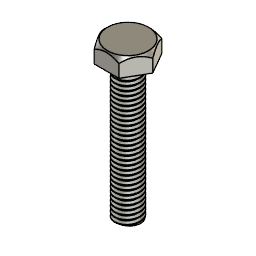
smartie_hopper_mechanism (Autodesk Fusion 360 archive; units mm, degrees)
design "M6 32 mm Hex Bolt"
part number: 2026-04-25-09-17-42-437
Autodesk Fusion 360 part; units mm, degrees
sketch "Thread" plane through (0, 0, 0) normal (0, 0, 1) x (1, 0, 0)
  circle A0 centre (0, 0) radius 3
  dimension "d2" = 6
  constraint coincident A0.centre origin
  measures "d2" diameter of A0
extrude "Extrude1" add sketch "Thread" along normal blind 32
sketch "Head" plane through (0, 0, 32) normal (0, 0, 1) x (-1, 0, 0)
  circle A0 centre (0, 0) radius 3
  line L0 (2.8868, -5) -> (5.7735, 0)
  line L1 (5.7735, 0) -> (2.8868, 5)
  line L2 (2.8868, 5) -> (-2.8868, 5)
  line L3 (-2.8868, 5) -> (-5.7735, 0)
  line L4 (-5.7735, 0) -> (-2.8868, -5)
  line L5 (-2.8868, -5) -> (2.8868, -5)
  dimension "d10" = 10
  constraint coincident A0.centre origin
  measures "d10" distance of L2 L5
extrude "Extrude2" add sketch "Head" along normal blind 4 contours A0 | L0 L1 L2 L3 L4 L5
thread "Thread1" "ISO Metric profile 6.0 M6x1 M6x1 6g" major diameter 5.884 minor diameter 4.7435 pitch 1 angle 60 modelled right hand crest width 0.1444 on face at (2.9963, -0.1495, 21.3333) crest through (2.942, 0, -0.25)
sketch "Head fillet" plane through (0, 0, 0) normal (0, 1, 0) x (1, 0, 0)
  line L0 (2.8868, -32) -> (5.7735, -32)
  line L1 (5.7735, -32) -> (5.7735, -36)
  line L2 (5.7735, -36) -> (2.8868, -36)
  line L3 (2.8868, -36) -> (2.8868, -32)
  line L4 (-5.7735, -32) -> (-2.8868, -32)
  line L5 (-2.8868, -32) -> (-2.8868, -36)
  line L6 (-2.8868, -36) -> (-5.7735, -36)
  line L7 (-5.7735, -36) -> (-5.7735, -32)
  line L8 (-2.8868, -32) -> (2.8868, -32)
  line L9 (2.8868, -32) -> (2.8868, -36)
  line L10 (2.8868, -36) -> (-2.8868, -36)
  line L11 (-2.8868, -36) -> (-2.8868, -32)
  line L12 (5.7735, -36) -> (4.7735, -36)
  line L13 (5.7735, -36) -> (5.7735, -35)
  line L14 (4.7735, -36) -> (5.7735, -35)
  dimension "d14" = 1
  dimension "d15" = 1
  constraint coincident L1.end L2.start
  constraint perpendicular L1 L12
  constraint perpendicular L2 L13
  measures "d14" distance of L1.end L12.end
  measures "d15" distance of L1.end L13.end
revolve "Revolve1" cut sketch "Head fillet" angle 360 about axis through (0, 0, 1.75) along (0, 0, 1) contours L1 L2 L12 L13 L14
equation "diameter = 6 mm" comment "An M6 hex bolt has a diameter of 6 mm."
equation "d2 = diameter"
equation "thread_height = 32 mm" comment "The length of the M6 hex bolt (excluding the head)."
equation "d4 = thread_height"
equation "head_height = 4 mm" comment "An M6 hex bolt has a head thickness of 4 mm."
equation "width_across_flats = 10 mm" comment "An M6 hex bolt has a width across the flats of 10 mm."
equation "d10 = width_across_flats"
equation "d11 = head_height"
equation "chamfer_side_length = 1 mm" comment "Chamfer on the top of the hex bolt head."
equation "d14 = chamfer_side_length"
equation "d15 = chamfer_side_length"
named bodies: "M6 32 mm Hex Bolt"

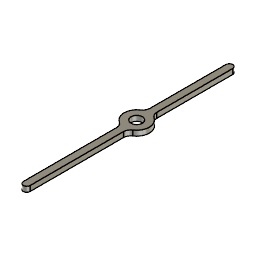
design "Mixer Arm"
part number: 2026-05-20-12-12-58-237
Autodesk Fusion 360 part; units mm, degrees
sketch "Mixer arm" plane through (0, 0, 0) normal (0, 0, 1) x (1, 0, 0)
  circle A0 centre (0, 0) radius 7.25
  circle A1 centre (0, 0) radius 3.25
  line L0 (-2, 55.25) -> (2, 55.25)
  line L1 (2, 55.25) -> (2, 3.25)
  line L2 (2, 3.25) -> (-2, 3.25)
  line L3 (-2, 3.25) -> (-2, 55.25)
  line L4 (-2, -3.25) -> (2, -3.25)
  line L5 (2, -3.25) -> (2, -65.25)
  line L6 (2, -65.25) -> (-2, -65.25)
  line L7 (-2, -65.25) -> (-2, -3.25)
  line L8 (-2, -7.25) -> (2, -7.25)
  line L9 (-2, 7.25) -> (2, 7.25)
  dimension "d3" = 6.5
  dimension "d5" = 14.5
  dimension "d6" = 2
  dimension "d7" = 2
  dimension "d8" = 2
  dimension "d9" = 2
  dimension "d14" = 58
  dimension "d15" = 48
  constraint coincident A0.centre A1.centre
  constraint concentric A0 A1
  constraint horizontal L0
  constraint vertical L1
  constraint horizontal L2
  constraint vertical L3
  constraint horizontal L4
  constraint vertical L5
  constraint horizontal L6
  constraint vertical L7
  constraint tangent A1 L2
  constraint tangent A1 L4
  constraint coincident L7 L8.start
  constraint coincident L5 L8.end
  constraint perpendicular L5 L8
  constraint tangent A0 L8
  constraint coincident L1 L9.end
  constraint perpendicular L1 L9
  constraint tangent A0 L9
  measures "d3" diameter of A1
  measures "d5" diameter of A0
  measures "d6" distance of A0.centre L1
  measures "d7" distance of A0.centre L3
  measures "d8" distance of A0.centre L7
  measures "d9" distance of A0.centre L5
  measures "d14" distance of L6 L8
  measures "d15" distance of L0 L9
extrude "Extrude1" add sketch "Mixer arm" along normal blind 3 contours A0 A1 L1 L2 L4 L5 | A0 L1 L2 L3 | A0 L1 L9 | A0 L5 L8 | A0 L4 L5 L7 | A0 L3 L9 | L0 L1 L3 L9 | A0 L7 L8 | L5 L6 L7 L8 | A0 A1 L2 L3 L4 L7
fillet "Fillet1" radius 4 4 edges at (2, -6.9687, 1.5) (2, 6.9687, 1.5) (-2, 6.9687, 1.5) (-2, -6.9687, 1.5)
fillet "Fillet2" radius 2 4 edges at (2, 55.25, 1.5) (-2, 55.25, 1.5) (-2, -65.25, 1.5) (2, -65.25, 1.5)
equation "stainless_steel_thickness = 3 mm" comment "The thickness of the 316 stainless steel sheets to laser cut."
equation "hole_diameter = 6.5 mm"
equation "d3 = hole_diameter"
equation "arm_thickness = 4 mm"
equation "d5 = hole_diameter + 2 * arm_thickness"
equation "d6 = arm_thickness / 2"
equation "d7 = arm_thickness / 2"
equation "d8 = arm_thickness / 2"
equation "d9 = arm_thickness / 2"
equation "d10 = stainless_steel_thickness"
equation "arm_length_front = 58 mm"
equation "arm_length_back = 48 mm"
equation "d14 = arm_length_front"
equation "d15 = arm_length_back"
equation "d17 = arm_thickness"
equation "d19 = arm_thickness / 2"
named bodies: "Mixer arm"

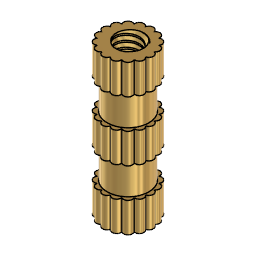
design "M2 10 mm Threaded Brass Insert"
part number: 2026-06-20-09-24-02-047
Autodesk Fusion 360 part; units mm, degrees
sketch "Brass thread outline" plane through (0, 0, 0) normal (0, 0, 1) x (1, 0, 0)
  circle A0 centre (0, 0) radius 1.4
  dimension "d4" = 2.8
  constraint coincident A0.centre origin
  measures "d4" diameter of A0
extrude "Extrude1" add sketch "Brass thread outline" along normal blind 10
sketch "Ridges" plane through (0, 0, 10) normal (0, 0, 1) x (-1, 0, 0)
  circle A0 centre (0, 0) radius 1.4
  circle A1 centre (0, 0) radius 1.7
  circle A2 centre (-0.0001, -1.4) radius 0.3
  circle A3 centre (0.5357, -1.2935) radius 0.3
  circle A4 centre (0.9899, -0.99) radius 0.3
  circle A5 centre (1.2934, -0.5358) radius 0.3
  circle A6 centre (1.4, -0.0001) radius 0.3
  circle A7 centre (1.2935, 0.5357) radius 0.3
  circle A8 centre (0.99, 0.9899) radius 0.3
  circle A9 centre (0.5358, 1.2934) radius 0.3
  circle A10 centre (0.0001, 1.4) radius 0.3
  circle A11 centre (-0.5357, 1.2935) radius 0.3
  circle A12 centre (-0.9899, 0.99) radius 0.3
  circle A13 centre (-1.2934, 0.5358) radius 0.3
  circle A14 centre (-1.4, 0.0001) radius 0.3
  circle A15 centre (-1.2935, -0.5357) radius 0.3
  circle A16 centre (-0.99, -0.9899) radius 0.3
  circle A17 centre (-0.5358, -1.2934) radius 0.3
  dimension "d8" = 3.4
  dimension "d29" = 0.0001
  dimension "d31" = 360
  constraint coincident A0.centre A1.centre
  constraint coincident A0 A2.centre
  constraint tangent A1 A2
  measures "d8" diameter of A1
  measures "d29" horizontal distance of A0.centre A2.centre
extrude "Extrude2" add sketch "Ridges" against normal blind 2 contours A0 A5 A6 A7 | A0 A5 A6 A7 | A0 A6 A7 | A0 A6 A7 | A0 A5 A6 | A0 A5 A6 | A0 A6 A7 A8 | A0 A6 A7 A8 | A2 A3 A4 A5 A6 A7 A8 A9 A10 A11 A12 A13 A14 A15 A16 A17 | A0 A4 A5 A6 | A0 A4 A5 A6 | A0 A7 A8 | A0 A7 A8 | A0 A7 A8 A9 | A0 A4 A5 | A0 A4 A5 | A0 A3 A4 A5 | A0 A7 A8 A9 | A0 A8 A9 A10 | A0 A8 A9 | A0 A3 A4 A5 | A0 A2 A3 A4 | A0 A3 A4 | A0 A8 A9 | A0 A8 A9 A10 | A0 A9 A10 A11 | A0 A9 A10 | A0 A3 A4 | A0 A2 A3 A17 | A0 A2 A3 | A0 A2 A3 A4 | A0 A9 A10 | A0 A9 A10 A11 | A0 A10 A11 A12 | A0 A10 A11 | A0 A2 A3 | A0 A2 A17 | A0 A2 A16 A17 | A0 A2 A3 A17 | A0 A10 A11 | A0 A10 A11 A12 | A0 A11 A12 A13 | A0 A11 A12 | A0 A2 A16 A17 | A0 A2 A17 | A0 A15 A16 A17 | A0 A16 A17 | A0 A11 A12 | A0 A11 A12 A13 | A0 A16 A17 | A0 A15 A16 A17 | A0 A12 A13 | A0 A12 A13 | A0 A12 A13 A14 | A0 A14 A15 A16 | A0 A15 A16 | A0 A15 A16 | A0 A12 A13 A14 | A0 A14 A15 A16 | A0 A13 A14 | A0 A13 A14 | A0 A13 A14 A15 | A0 A13 A14 A15 | A0 A14 A15 | A0 A14 A15
pattern_linear "R-Pattern1" count 3 spacing 4 along (0, 0, -1) of "Extrude2"
sketch "Thread hole" plane through (0, 0, 10) normal (0, 0, 1) x (-1, 0, 0)
  circle A0 centre (0, 0) radius 1
  arc A1 (0.292, -1.4685) -> (0.8317, -1.2449) centre (0.5357, -1.2935) ccw
  arc A2 (0.8317, -1.2449) -> (1.2448, -0.8319) centre (0.9899, -0.99) ccw
  arc A3 (1.2448, -0.8319) -> (1.4684, -0.2922) centre (1.2934, -0.5358) ccw
  arc A4 (1.4684, -0.2922) -> (1.4685, 0.292) centre (1.4, -0.0001) ccw
  arc A5 (1.4685, 0.292) -> (1.2449, 0.8317) centre (1.2935, 0.5357) ccw
  arc A6 (1.2449, 0.8317) -> (0.8319, 1.2448) centre (0.99, 0.9899) ccw
  arc A7 (0.8319, 1.2448) -> (0.2922, 1.4684) centre (0.5358, 1.2934) ccw
  arc A8 (0.2922, 1.4684) -> (-0.292, 1.4685) centre (0.0001, 1.4) ccw
  arc A9 (-0.292, 1.4685) -> (-0.8317, 1.2449) centre (-0.5357, 1.2935) ccw
  arc A10 (-0.8317, 1.2449) -> (-1.2448, 0.8319) centre (-0.9899, 0.99) ccw
  arc A11 (-1.2448, 0.8319) -> (-1.4684, 0.2922) centre (-1.2934, 0.5358) ccw
  arc A12 (-1.4684, 0.2922) -> (-1.4685, -0.292) centre (-1.4, 0.0001) ccw
  arc A13 (-1.4685, -0.292) -> (-1.2449, -0.8317) centre (-1.2935, -0.5357) ccw
  arc A14 (-1.2449, -0.8317) -> (-0.8319, -1.2448) centre (-0.99, -0.9899) ccw
  arc A15 (-0.8319, -1.2448) -> (-0.2922, -1.4684) centre (-0.5358, -1.2934) ccw
  arc A16 (-0.2922, -1.4684) -> (0.292, -1.4685) centre (-0.0001, -1.4) ccw
  dimension "d11" = 2
  constraint coincident A0.centre origin
  measures "d11" diameter of A0
extrude "Extrude3" cut sketch "Thread hole" against normal blind 10 contours A0
thread "Thread1" "ISO Metric profile 2.0 M2x0.4 M2x0.4 6H" major diameter 2.074 minor diameter 1.623 pitch 0.4 angle 60 modelled right hand crest width 0.1065 on face at (-0.9988, 0.0498, 3.3333) crest through (-0.8115, 0, 9.9)
equation "outer_diameter = 2.8 mm" comment "The outer diameter of the non-ridged parts."
equation "hole_diameter = 2 mm" comment "The thread diameter of the brass insert. 2 mm for this M2 insert."
equation "height = 10 mm" comment "The height of the brass thread insert. 10 mm for this model."
equation "d4 = outer_diameter"
equation "d5 = height"
equation "ridge_diameter = 3.4 mm" comment "The outer diameter of the ridged parts."
equation "d8 = ridge_diameter"
equation "d9 = -ridge_height"
equation "d11 = hole_diameter"
equation "d12 = -height"
equation "number_of_ridges = 3" comment "The number of ridges to have along the outside."
equation "d23 = number_of_ridges"
equation "d25 = -ridge_pattern_length"
equation "ridge_pattern_length = height - ridge_height" comment "The distance to use for the rectangular pattern that repeats the ridges."
equation "ridge_height = 2 mm" comment "The height of the individual ridges."
named bodies: "M2 10 mm Threaded Brass Insert"

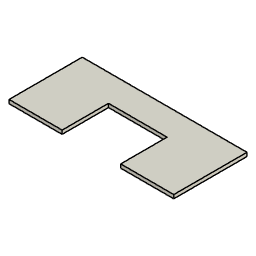
design "Colour Detection Mechanism Top Panel"
part number: 2025-05-13-09-48-31-121
Autodesk Fusion 360 part; units mm, degrees
sketch "Sorting Mechanism Top Panel" plane through (0, 0, 0) normal (0, 0, 1) x (1, 0, 0)
  line L0 (0, 0) -> (270, 0)
  line L1 (270, 0) -> (270, 120)
  line L2 (270, 120) -> (0, 120)
  line L3 (0, 120) -> (0, 0)
  dimension "d1" = 270
  dimension "d2" = 120
  constraint horizontal L0
  constraint vertical L1
  constraint horizontal L2
  constraint vertical L3
  constraint coincident L0.start L3.end
  measures "d1" distance of L0.start L0.end
  measures "d2" distance of L0.end L1.end
extrude "Extrude1" add sketch "Sorting Mechanism Top Panel" along normal blind 6
sketch "Smartie Hopper Hole" plane through (0, 0, 6) normal (0, 0, 1) x (-1, 0, 0)
  line L0 (0, -120) -> (0, 0)
  line L1 (0, 0) -> (-270, 0)
  line L2 (-270, 0) -> (-270, -120)
  line L3 (-270, -120) -> (0, -120)
  line L4 (-87, -76) -> (-183, -76)
  line L5 (-183, -76) -> (-183, 0)
  line L6 (-183, 0) -> (-87, 0)
  line L7 (-87, 0) -> (-87, -76)
  dimension "d7" = 96
  dimension "d9" = 76
  dimension "d10" = 87
  dimension "d11" = 87
  constraint horizontal L4
  constraint vertical L5
  constraint horizontal L6
  constraint vertical L7
  constraint collinear L1 L6
  measures "d7" distance of L4.start L4.end
  measures "d9" distance of L4.end L5.end
  measures "d10" distance of L0 L7
  measures "d11" distance of L2 L5
extrude "Extrude2" cut sketch "Smartie Hopper Hole" against normal blind 6 contours L1 L4 L5 L6 L7
equation "d3 = MDF_thickness"
equation "acrylic_thickness = 3 mm" comment "Thickness of the clear acrylic panels"
equation "MDF_thickness = 6 mm" comment "Thickness of the MDF panels"
equation "d7 = smarties_hopper_width + 2 * acrylic_thickness"
equation "smarties_hopper_width = 90 mm" comment "Width of the Smarties hopper"
equation "d9 = smarties_hopper_depth + 2 * acrylic_thickness"
equation "d10 = ( 270 mm - ( smarties_hopper_width + 2 * acrylic_thickness ) ) / 2"
equation "d14 = -MDF_thickness"
equation "smarties_hopper_depth = 70 mm" comment "Depth of the Smarties hopper"
named bodies: "Sorting Mechanism Top Panel"
